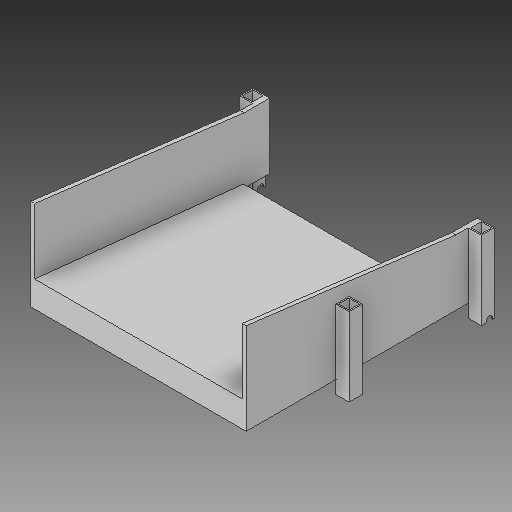
# Autodesk Inventor part: hopper_bottom2
Saved by Autodesk Inventor 2017 (Build 210142000, 142)
## iProperties
Created: 2020-01-18
Part Number: hopper_bottom2
Material: Generic
Document SubType Name: Modeling
Designer: S338578040
Density: 1 g/cm^3
Appearance: Default
Author: S338578040
Autodesk Inventor part; units mm, degrees
ref_plane "YZ Plane" through (0, 0, 0) normal (1, 0, 0) x (0, 1, 0)
ref_plane "XZ Plane" through (0, 0, 0) normal (0, 1, 0) x (-1, 0, 0)
ref_plane "XY Plane" through (0, 0, 0) normal (0, 0, 1) x (1, 0, 0)
sketch "Sketch1" plane through (0, 0, 0) normal (0, 1, 0) x (-1, 0, 0)
  line L0 (0, 0) -> (-403.86, 0)
  line L1 (-403.86, 0) -> (-403.86, -406.4)
  line L2 (-403.86, -406.4) -> (0, -406.4)
  line L3 (0, -406.4) -> (0, 0)
  dimension "d0" = 406.4
  dimension "d1" = 403.86
  constraints: 8 end point, 2 parallel, 1 horizontal, 1 perpendicular
  measures "d0" distance of L2.end L0.start
  measures "d1" distance of L0.start L0.end
extrude "Extrusion1" add sketch "Sketch1" along normal blind 7.62
sketch "Sketch2" plane through (403.86, 0, 0) normal (1, 0, 0) x (0, 0, -1)
  line L0 (0, 0) -> (406.4, 0) projected
  line L1 (0, 0) -> (406.4, 0)
  line L2 (406.4, 0) -> (406.4, 127)
  line L3 (406.4, 127) -> (0, 127)
  line L4 (0, 127) -> (0, 0)
  dimension "d4" = 127
  constraints: 8 end point, 2 parallel, 1 horizontal, 1 perpendicular
  measures "d4" distance of L3.end L0.start
extrude "Extrusion2" add sketch "Sketch2" along normal blind 7.62
sketch "Sketch3" plane through (0, 0, -406.4) normal (-1, 0, 0) x (0, 0, 1)
  line L0 (0, 0) -> (0, 7.62) projected
  line L1 (406.4, 127) -> (406.4, 7.62) projected
  line L2 (0, 0) -> (406.4, 0)
  line L3 (406.4, 0) -> (406.4, 127)
  line L4 (406.4, 127) -> (0, 127)
  line L5 (0, 127) -> (0, 0)
  point P0 (406.4, 0)
  constraints: 8 end point, 2 parallel, 1 horizontal, 1 perpendicular
extrude "Extrusion3" add sketch "Sketch3" along normal blind 7.62
sketch "Sketch6" plane through (403.86, 7.62, -406.4) normal (0, 0, -1) x (-1, 0, 0)
  line L0 (-7.62, 119.38) -> (414.02, 119.38) projected
  line L1 (-7.62, 119.38) -> (0, 119.38)
  line L2 (0, 119.38) -> (0, -33.02)
  line L3 (0, -33.02) -> (-7.62, -33.02)
  line L4 (-7.62, -33.02) -> (-7.62, 119.38)
  point P0 (403.86, -7.62)
  dimension "d14" = 152.4
  constraints: 8 end point, 2 parallel, 1 horizontal, 1 perpendicular
  measures "d14" distance of L1.end L2.end
extrude "Extrusion6" add sketch "Sketch6" along normal blind 50.8
sketch "Sketch7" plane through (0, 7.62, -406.4) normal (0, 0, -1) x (-1, 0, 0)
  line L0 (-406.4, 119.38) -> (0, 119.38) projected
  line L1 (0, 119.38) -> (7.62, 119.38)
  line L2 (7.62, 119.38) -> (7.62, -33.02)
  line L3 (7.62, -33.02) -> (0, -33.02)
  line L4 (0, -33.02) -> (0, 119.38)
  point P0 (0, -7.62)
  dimension "d17" = 152.4
  constraints: 8 end point, 2 parallel, 1 horizontal, 1 perpendicular
  measures "d17" distance of L1.end L2.end
extrude "Extrusion7" add sketch "Sketch7" along normal blind 50.8
sketch "Sketch14" plane through (403.86, 0, 0) normal (-1, 0, 0) x (0, 0, 1)
  line L0 (0, 0) -> (-406.4, 0) projected
  line L1 (0, 0) -> (0, 50.8)
  line L2 (0, 127) -> (0, 7.62) projected
  line L3 (-406.4, 0) -> (-406.4, 7.62) projected
  line L4 (0, 50.8) -> (-406.4, 7.62)
  line L5 (0, 7.62) -> (-406.4, 7.62) projected
  line L6 (-406.4, 7.62) -> (0, 7.62)
  line L7 (0, 7.62) -> (0, 50.8)
  dimension "d45" = 50.8
  constraints: 8 end point, 2 collinear, 1 point on line
  measures "d45" distance of L0.start L1.end
extrude "Extrusion14" add sketch "Sketch14" along normal blind 403.86 contours L5 L4 L1
sketch "Sketch15" plane through (403.86, 0, 0) normal (-1, 0, 0) x (0, 0, 1)
  line L0 (0, 0) -> (0, 127) projected
  line L1 (0, 127) -> (0, 177.8)
  line L2 (0, 177.8) -> (-407.7581, 127)
  line L3 (0, 127) -> (-457.2, 127) projected
  line L4 (0, 127) -> (-407.7581, 127)
  dimension "d48" = 50.8
  constraints: 6 end point, 1 perpendicular, 1 point on line, 1 vertical
  measures "d48" distance of L0.end L1.end
extrude "Extrusion15" add sketch "Sketch15" against normal blind 7.62
sketch "Sketch16" plane through (-7.62, 0, -406.4) normal (-1, 0, 0) x (0, 0, 1)
  line L0 (406.4, 127) -> (-50.8, 127) projected
  line L1 (406.4, 50.8) -> (406.4, 177.8) projected
  line L2 (406.4, 127) -> (406.4, 177.8)
  line L3 (406.4, 177.8) -> (-1.3581, 127) projected
  line L4 (406.4, 177.8) -> (-1.3581, 127)
  line L5 (-1.3581, 127) -> (406.4, 127)
  point P0 (406.4, 0)
  constraints: 6 end point, 2 collinear, 1 perpendicular
extrude "Extrusion16" add sketch "Sketch16" against normal blind 7.62
sketch "Sketch17" plane through (403.86, 127, -457.2) normal (0, 1, 0) x (1, 0, 0)
  line L0 (-411.48, -49.4419) -> (-411.48, 0) projected
  line L1 (-411.48, 0) -> (-436.88, 0)
  line L2 (-436.88, 0) -> (-436.88, -25.4)
  line L3 (-436.88, -25.4) -> (-411.48, -25.4)
  line L4 (-411.48, -25.4) -> (-411.48, 0)
  line L5 (-434.34, -2.54) -> (-414.02, -2.54)
  line L6 (-414.02, -2.54) -> (-414.02, -22.86)
  line L7 (-414.02, -22.86) -> (-434.34, -22.86)
  line L8 (-434.34, -22.86) -> (-434.34, -2.54)
  line L9 (7.62, 0) -> (33.02, 0)
  line L10 (33.02, 0) -> (33.02, -25.4)
  line L11 (33.02, -25.4) -> (7.62, -25.4)
  line L12 (7.62, -25.4) -> (7.62, 0)
  line L13 (10.16, -22.86) -> (30.48, -22.86)
  line L14 (30.48, -22.86) -> (30.48, -2.54)
  line L15 (30.48, -2.54) -> (10.16, -2.54)
  line L16 (10.16, -2.54) -> (10.16, -22.86)
  point P0 (-403.86, -457.2)
  dimension "d53" = 25.4
  dimension "d54" = 25.4
  dimension "d55" = 2.54
  dimension "d56" = 25.4
  dimension "d57" = 25.4
  dimension "d58" = 2.54
  constraints: 32 end point, 8 parallel, 4 perpendicular, 2 horizontal, 6 other
  measures "d53" distance of L3.end L2.end
  measures "d54" distance of L2.end L1.end
  measures "d55" distance between parallel lines of L1 L5
  measures "d56" distance of L10.end L11.end
  measures "d57" distance of L9.end L10.end
  measures "d58" distance between parallel lines of L11 L13
extrude "Extrusion17" add sketch "Sketch17" against normal blind 152.4
sketch "Sketch18" plane through (403.86, 7.62, -457.2) normal (0, 0, -1) x (-1, 0, 0)
  line L0 (403.86, 119.38) -> (403.86, -33.02) projected
  line L1 (411.48, -33.02) -> (403.86, -33.02) projected
  line L2 (403.86, -33.02) -> (411.48, -33.02)
  line L3 (411.48, -7.62) -> (411.48, -33.02) projected
  line L4 (411.48, -33.02) -> (411.48, -7.62)
  line L5 (411.48, -7.62) -> (403.86, -7.62)
  line L6 (403.86, -33.02) -> (403.86, -7.62)
  line L7 (0, -33.02) -> (0, 119.38) projected
  line L8 (0, -33.02) -> (-7.62, -33.02)
  line L9 (0, -33.02) -> (-33.02, -33.02) projected
  line L10 (-7.62, -33.02) -> (-7.62, -7.62)
  line L11 (-7.62, -7.62) -> (0, -7.62)
  line L12 (0, -7.62) -> (0, -33.02)
  dimension "d61" = 7.62
  dimension "d62" = 7.62
  constraints: 16 end point, 4 perpendicular, 3 point on line, 1 collinear, 1 horizontal
  measures "d61" distance of L0.end L1.start
  measures "d62" distance of L7.start L8.end
extrude "Extrusion18" cut sketch "Sketch18" against normal blind 63.5
sketch "Sketch19" plane through (-7.62, 127, -407.7581) normal (0, 1, 0) x (1, 0, 0)
  line L0 (-2.54, -210.2731) -> (-22.86, -210.2731) projected
  line L1 (-25.4, -207.7331) -> (0, -207.7331) projected
  line L2 (-2.54, -230.5931) -> (-2.54, -210.2731) projected
  line L3 (-25.4, -233.1331) -> (0, -233.1331) projected
  line L4 (-22.86, -230.5931) -> (-2.54, -230.5931) projected
  line L5 (-25.4, -207.7331) -> (-25.4, -233.1331) projected
  line L6 (-22.86, -210.2731) -> (-22.86, -230.5931) projected
  line L7 (0, -207.7331) -> (-25.4, -207.7331)
  line L8 (-25.4, -207.7331) -> (-25.4, -233.1331)
  line L9 (-25.4, -233.1331) -> (0, -233.1331)
  line L10 (0, -233.1331) -> (0, -207.7331)
  line L11 (-2.54, -210.2731) -> (-22.86, -210.2731)
  line L12 (-22.86, -210.2731) -> (-22.86, -230.5931)
  line L13 (-22.86, -230.5931) -> (-2.54, -230.5931)
  line L14 (-2.54, -230.5931) -> (-2.54, -210.2731)
  line L15 (419.1, -233.1331) -> (444.5, -233.1331) projected
  line L16 (444.5, -233.1331) -> (444.5, -207.7331) projected
  line L17 (419.1, -207.7331) -> (444.5, -207.7331) projected
  line L18 (419.1, -233.1331) -> (419.1, -207.7331) projected
  line L19 (421.64, -210.2731) -> (441.96, -210.2731) projected
  line L20 (441.96, -210.2731) -> (441.96, -230.5931) projected
  line L21 (441.96, -230.5931) -> (421.64, -230.5931) projected
  line L22 (421.64, -230.5931) -> (421.64, -210.2731) projected
  line L23 (444.5, -207.7331) -> (419.1, -207.7331)
  line L24 (419.1, -207.7331) -> (419.1, -233.1331)
  line L25 (419.1, -233.1331) -> (444.5, -233.1331)
  line L26 (444.5, -233.1331) -> (444.5, -207.7331)
  line L27 (441.96, -210.2731) -> (421.64, -210.2731)
  line L28 (421.64, -210.2731) -> (421.64, -230.5931)
  line L29 (421.64, -230.5931) -> (441.96, -230.5931)
  line L30 (441.96, -230.5931) -> (441.96, -210.2731)
  point P0 (7.62, -407.7581)
  constraints: 32 end point, 8 parallel, 4 horizontal, 4 perpendicular
extrude "Extrusion19" add sketch "Sketch19" against normal blind 152.4
sketch "Sketch20" plane through (436.88, 127, -431.8) normal (1, 0, 0) x (0, 0, -1)
  circle A0 centre (15.6875, -150.0895) radius 6.35 projected
  circle A1 centre (12.7, -141.5035) radius 6.35
  point P0 (-431.8, -127)
  dimension "d67" = 12.7
  constraints: 1 centre point
  measures "d67" diameter of A1
extrude "Extrusion20" cut sketch "Sketch20" against normal blind 530.225 contours A0 A1 | A1 A0 picked at (16.199, -153.3641) picked at (14.6075, -146.2758)
sketch "Sketch21" plane through (-7.62, 0, -406.4) normal (-1, 0, 0) x (0, 0, 1)
  line L0 (-25.4, 0) -> (-25.4, -25.4) projected
  line L1 (-25.4, 0) -> (0, 0)
  line L2 (0, 0) -> (0, 25.4)
  line L3 (0, 25.4) -> (-25.4, 25.4)
  line L4 (-25.4, 25.4) -> (-25.4, 0)
  point P0 (406.4, 0)
  dimension "d70" = 25.4
  dimension "d71" = 25.4
  constraints: 8 end point, 2 parallel, 1 horizontal, 1 perpendicular
  measures "d70" distance of L3.end L2.end
  measures "d71" distance of L2.end L1.end
extrude "Extrusion21" add sketch "Sketch21" along normal blind 25.4
sketch "Sketch22" plane through (-33.02, 127, -457.2) normal (-1, 0, 0) x (0, 0, 1)
  circle A0 centre (27.6854, -132.1414) radius 2.0193 projected
  point P0 (457.2, -127)
extrude "Extrusion22" cut sketch "Sketch22" against normal blind 127
body "Solid1"
